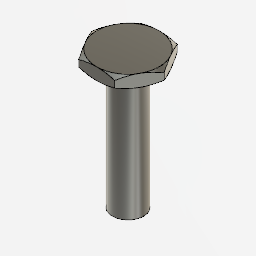
Hex_Bolt (Autodesk Fusion 360 design; units mm, degrees)
Autodesk Fusion 360 part; units mm, degrees
sketch "Sketch1" plane through (0, 0, 0) normal (0, 0, 1) x (1, 0, 0)
  line L0 (-3.6662, -6.35) -> (3.6662, -6.35)
  line L1 (3.6662, -6.35) -> (7.3323, 0)
  line L2 (7.3323, 0) -> (3.6662, 6.35)
  line L3 (3.6662, 6.35) -> (-3.6662, 6.35)
  line L4 (-3.6662, 6.35) -> (-7.3323, 0)
  line L5 (-7.3323, 0) -> (-3.6662, -6.35)
  dimension "hexwidth" = 12.7
  measures "hexwidth" distance of L0 L3
extrude "Extrude1" add sketch "Sketch1" along normal blind 2.4638
sketch "Sketch2" plane through (0, 0, 0) normal (0, 0, -1) x (1, 0, 0)
  line L0 (-3.6662, 6.35) -> (-7.3323, 0)
  line L1 (-7.3323, 0) -> (-3.6662, -6.35)
  line L2 (-3.6662, -6.35) -> (3.6662, -6.35)
  line L3 (3.6662, -6.35) -> (7.3323, 0)
  line L4 (7.3323, 0) -> (3.6662, 6.35)
  line L5 (3.6662, 6.35) -> (-3.6662, 6.35)
  circle A0 centre (0, 0) radius 3.175
  dimension "diameter" = 6.35
  measures "diameter" diameter of A0
extrude "Extrude2" add sketch "Sketch2" along normal blind 25.4 contours A0
sketch "Sketch3" plane through (0, 0, 2.4638) normal (0, 0, 1) x (-1, 0, 0)
  line L0 (7.3323, 0) -> (3.6662, 6.35) construction
  line L1 (3.6662, 6.35) -> (-3.6662, 6.35) construction
  line L2 (-3.6662, 6.35) -> (-7.3323, 0) construction
  line L3 (-7.3323, 0) -> (-3.6662, -6.35) construction
  line L4 (-3.6662, -6.35) -> (3.6662, -6.35) construction
  line L5 (3.6662, -6.35) -> (7.3323, 0) construction
  circle A0 centre (0, 0) radius 6.35
  circle A1 centre (0, 0) radius 19.05
  dimension "d9" = 12.7
  measures "d9" distance of A0 A1
extrude "Extrude4" cut sketch "Sketch3" against normal blind 2.032 draft -60
sketch "Sketch4" plane through (0, 0, 0) normal (0, 0, -1) x (1, 0, 0)
  circle A0 centre (0, 0) radius 3.175
  line L0 (-3.6662, 6.35) -> (-7.3323, 0) construction
  line L1 (-7.3323, 0) -> (-3.6662, -6.35) construction
  line L2 (-3.6662, -6.35) -> (3.6662, -6.35) construction
  line L3 (3.6662, -6.35) -> (7.3323, 0) construction
  line L4 (7.3323, 0) -> (3.6662, 6.35) construction
  line L5 (3.6662, 6.35) -> (-3.6662, 6.35) construction
  circle A1 centre (0, 0) radius 6.35
  circle A2 centre (0, 0) radius 19.05
  dimension "d12" = 12.7
  measures "d12" distance of A1 A2
extrude "Extrude5" cut sketch "Sketch4" against normal blind 2.032 draft -60 contours A2
equation "heightmax = 0.097 in"
equation "length = 1.0 in"
equation "hexcut2 = -0.08 in"
equation "hexcut1 = -0.08 in"
